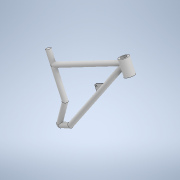
# Autodesk Inventor part: 車架
Saved by Autodesk Inventor 2020 (Build 240168000, 168)
## iProperties
Created: 2021-05-19
Part Number: 車架
Material: 一般
Document SubType Name: Modeling
Designer: 林昱秀
Density: 1 g/cm^3
Appearance: 預設
Author: 林昱秀
Autodesk Inventor part; units mm, degrees
sketch "草圖2" plane through (0, 0, 0) normal (0, 0, 1) x (1, 0, 0)
  line L0 (0, 0) -> (2326.9129, -0.931) construction
  line L1 (2326.9129, -0.931) -> (2326.3916, -1303.9311) construction
  line L2 (2326.3916, -1303.9311) -> (-0.5213, -1303.0001) construction
  line L3 (-0.5213, -1303.0001) -> (0, 0) construction
  line L4 (720.5949, -946.6697) -> (786.7892, -914.8619)
  line L5 (672.9691, -624.7758) -> (1152.635, -373.5516)
  line L6 (669.6641, -806.0741) -> (1364.2388, -806.0741)
  line L7 (710.8785, -951.3386) -> (545.7785, -356.0073)
  line L8 (1180.3272, -432.9379) -> (1140.1785, -346.8386)
  line L9 (710.8785, -951.3386) -> (710.8785, -1299.3386)
  line L10 (638.4216, -549.3614) -> (751.3073, -795.7819)
  line L11 (751.3073, -795.7819) -> (713.5901, -940.9053)
  line L12 (786.7892, -914.8619) -> (1136.3124, -397.7027)
  line L13 (951.5937, -605.2362) -> (968.6017, -645.8497)
  line L14 (956.0469, -592.5848) -> (1032.735, -550.9573)
  circle A0 centre (960.8177, -601.3736) radius 5
  arc A1 (713.5901, -940.9053) -> (720.5949, -946.6697) centre (718.4293, -942.163) ccw
  line L15 (271.3556, -930.1858) -> (649.2771, -969.8768)
  line L16 (726.1503, -692.8447) -> (649.2771, -969.8768)
  line L17 (726.1503, -692.8447) -> (271.3556, -930.1858)
  line L18 (649.2771, -969.8768) -> (673.3417, -883.1537)
  line L19 (673.3417, -883.1537) -> (271.3556, -930.1858)
  line L20 (678.9646, -885.9308) -> (725.6462, -880.4691)
  arc A2 (956.0469, -592.5848) -> (951.5937, -605.2362) centre (960.8175, -601.3735) ccw
  line L21 (1136.3124, -397.7027) -> (1142.6218, -394.671)
  point P0 (949.8477, -601.0669)
  point P1 (952.0743, -594.7412)
  point P2 (960.8175, -601.3735)
  point P3 (960.8175, -601.3735)
  dimension "d18" = 65
  dimension "d24" = 95
  dimension "d27" = 604.5
  dimension "d28" = 594.4
  dimension "d29" = 348
  dimension "d41" = 429.3
  dimension "d43" = 674.5628
  dimension "d71" = 10
  dimension "d92" = 5
  dimension "d106" = 74.5
  dimension "d107" = 31.354
  dimension "d131" = 393.7
  dimension "d133" = 380
  dimension "d135" = 513
  dimension "d136" = 287.5
  dimension "d138" = 90
  dimension "d140" = 47
  dimension "d144" = 10
  dimension "d145" = 10
  dimension "d167" = 7
  constraints: 36 end point, 7 point on line, 4 point on circle, 4 tangent, 3 centre point, 1 horizontal, 1 vertical, 6 other
  measures "d18" angle of L6 L8
  measures "d24" distance of L8.start L8.end
  measures "d27" vertical distance of L7.start L8.end
  measures "d28" horizontal distance of L7.end L8.end
  measures "d29" distance of L7.start L9.end
  measures "d41" horizontal distance of L8.end L7.start
  measures "d43" vertical distance of L5.start L9.end
  measures "d71" diameter of A0
  measures "d92" radius of A1
  measures "d106" angle of L6 L7
  measures "d107" distance from line of L12 A0.centre
  measures "d131" distance from line of L4 L10.start
  measures "d133" distance of L15.start L15.end
  measures "d135" distance of L17.start L15.start
  measures "d136" distance of L16.start L15.end
  measures "d138" distance of L15.end L18.end
  measures "d140" distance of L20.end L20.start
  measures "d144" radius of A2
  measures "d145" radius of A2
  measures "d167" distance of L21.end L12.end
ref_plane "工作平面2" through (672.9691, -624.7758, 0) normal (0.8859, 0.464, 0) x (-0.464, 0.8859, 0)
sketch "草圖4" plane through (672.9691, -624.7758, 0) normal (0.8859, 0.464, 0) x (-0.464, 0.8859, 0)
  circle A0 centre (0, 0) radius 15
  point P0 (865.6938, 0)
  dimension "d44" = 30
  constraints: 1 centre point
  measures "d44" diameter of A0
sweep "掃掠1" add profiles "草圖4" path "草圖2" path curves L5
ref_plane "工作平面3" through (638.4216, -549.3614, 0) normal (0.4165, -0.9091, 0) x (0.9091, 0.4165, 0)
sketch "草圖5" plane through (638.4216, -549.3614, 0) normal (0.4165, -0.9091, 0) x (0.9091, 0.4165, 0)
  circle A0 centre (0, 0) radius 15
  point P0 (-351.6187, 0)
  dimension "d47" = 30
  constraints: 1 centre point
  measures "d47" diameter of A0
sweep "掃掠2" add profiles "草圖5" path "草圖2" separate body path curves L10 L11 A1 L4 L12 L21
ref_plane "工作平面4" through (1140.1785, -346.8386, 0) normal (-0.4226, 0.9063, 0) x (-0.9063, -0.4226, 0)
sketch "草圖6" plane through (1140.1785, -346.8386, 0) normal (-0.4226, 0.9063, 0) x (-0.9063, -0.4226, 0)
  circle A0 centre (0, 0) radius 17.5
  circle A1 centre (0, 0) radius 30
  point P0 (886.7723, 0)
  dimension "d50" = 35
  dimension "d51" = 60
  constraints: 2 centre point, 1 coincident
  measures "d50" diameter of A0
  measures "d51" diameter of A1
extrude "擠出1" add sketch "草圖6" against normal blind 95 contours A0 | A1 bodies 1
extrude "擠出2" cut sketch "草圖6" against normal blind 95 contours A0 bodies 1
extrude "擠出3" add sketch "草圖2" along normal mid plane 5 contours L13 A2 L14 L12 bodies 1
